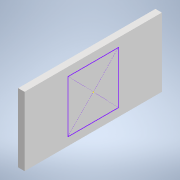
# Autodesk Inventor part: NASA-20-MM-MP-01
Saved by Autodesk Inventor 2020 (Build 240168000, 168)
## iProperties
Created: 2019-09-22
Part Number: NASA-20-MM-MP-01
Material: Aluminum 6061
Document SubType Name: Modeling
Designer: Rick Szalay
Density: 2.7 g/cm^3
Appearance: Aluminum - Flat
Author: Rick Szalay
Autodesk Inventor part; units mm, degrees
ref_plane "YZ Plane" through (0, 0, 0) normal (1, 0, 0) x (0, 1, 0)
ref_plane "XZ Plane" through (0, 0, 0) normal (0, 1, 0) x (-1, 0, 0)
ref_plane "XY Plane" through (0, 0, 0) normal (0, 0, 1) x (1, 0, 0)
sketch "Sketch1" plane through (0, 0, 0) normal (1, 0, 0) x (0, 1, 0)
  line L0 (-25.4, -50.8) -> (25.4, -50.8)
  line L1 (25.4, -50.8) -> (25.4, 50.8)
  line L2 (25.4, 50.8) -> (-25.4, 50.8)
  line L3 (-25.4, 50.8) -> (-25.4, -50.8)
  line L4 (-25.4, -50.8) -> (25.4, 50.8) construction
  line L5 (25.4, -50.8) -> (-25.4, 50.8) construction
  point P0 (0, 0)
  dimension "d0" = 50.8
  dimension "d1" = 101.6
  constraints: 12 end point, 2 midpoint, 2 parallel, 1 horizontal, 1 perpendicular
  measures "d0" distance of L0.start L0.end
  measures "d1" distance between parallel lines of L2 L0
extrude "Extrusion1" add sketch "Sketch1" along normal blind 57.15
fillet "Fillet2" radius 6.35 4 edges at (28.575, 25.4, 50.8) (28.575, -25.4, 50.8) (28.575, -25.4, -50.8) (28.575, 25.4, -50.8)
sketch "Sketch5" plane through (57.15, 0, 0) normal (1, 0, 0) x (0, 0, -1)
  arc A0 (50.8, 19.05) -> (44.45, 25.4) centre (44.45, 19.05) ccw projected
  line L0 (44.45, 25.4) -> (-44.45, 25.4) projected
  arc A1 (-44.45, 25.4) -> (-50.8, 19.05) centre (-44.45, 19.05) ccw projected
  line L1 (-50.8, 19.05) -> (-50.8, -19.05) projected
  arc A2 (-50.8, -19.05) -> (-44.45, -25.4) centre (-44.45, -19.05) ccw projected
  line L2 (-44.45, -25.4) -> (44.45, -25.4) projected
  arc A3 (44.45, -25.4) -> (50.8, -19.05) centre (44.45, -19.05) ccw projected
  line L3 (50.8, -19.05) -> (50.8, 19.05) projected
  point P0 (0, 0)
hole "Hole2" at (57.15, -19.05, -44.45) at (57.15, -19.05, 44.45) at (57.15, 19.05, 44.45) at (57.15, 19.05, -44.45) direction (-1, 0, 0) diameter 6.7564 end through all clearance for "Flat Head Machine Screw (82)" size "1/4" standard "Ansi Unified Screw Threads"
sketch "Sketch6" plane through (57.15, 0, 0) normal (1, 0, 0) x (0, 0, -1)
  circle A0 centre (44.45, -19.05) radius 3.3782 projected
  circle A1 centre (44.45, -19.05) radius 6.35
  circle A2 centre (44.45, 19.05) radius 3.3782 projected
  circle A3 centre (44.45, 19.05) radius 6.35
  circle A4 centre (-44.45, 19.05) radius 3.3782 projected
  circle A5 centre (-44.45, 19.05) radius 6.35
  circle A6 centre (-44.45, -19.05) radius 3.3782 projected
  circle A7 centre (-44.45, -19.05) radius 6.35
  line L0 (-46.99, 21.59) -> (46.99, 21.59)
  line L1 (46.99, 21.59) -> (46.99, -21.59)
  line L2 (46.99, -21.59) -> (-46.99, -21.59)
  line L3 (-46.99, -21.59) -> (-46.99, 21.59)
  line L4 (-46.99, 21.59) -> (46.99, -21.59) construction
  line L5 (46.99, 21.59) -> (-46.99, -21.59) construction
  arc A8 (44.45, -25.4) -> (50.8, -19.05) centre (44.45, -19.05) ccw projected
  arc A9 (50.8, 19.05) -> (44.45, 25.4) centre (44.45, 19.05) ccw projected
  arc A10 (-44.45, 25.4) -> (-50.8, 19.05) centre (-44.45, 19.05) ccw projected
  arc A11 (-50.8, -19.05) -> (-44.45, -25.4) centre (-44.45, -19.05) ccw projected
  line L6 (50.8, -19.05) -> (50.8, 19.05) projected
  point P0 (0, 0)
  point P1 (-46.99, 13.2301)
  point P2 (-46.99, -13.2301)
  point P3 (-38.6301, -21.59)
  point P4 (38.6301, -21.59)
  point P5 (46.99, -13.2301)
  point P6 (46.99, 13.2301)
  point P7 (38.6301, 21.59)
  point P8 (-38.6301, 21.59)
  dimension "d23" = 43.18
  dimension "d24" = 3.81
  constraints: 12 end point, 8 concentric, 4 centre point, 3 coincident, 2 midpoint, 2 parallel, 1 horizontal, 1 perpendicular
  measures "d23" distance of L0.end L1.end
  measures "d24" distance between parallel lines of L6 L1
extrude "Extrusion2" cut sketch "Sketch6" against normal through all contours A1 L2 A7 L3 A5 L0 A3 L1
fillet "Fillet3" radius 3.175 8 edges at (28.575, 13.2301, 46.99) (28.575, 21.59, 38.6301) (28.575, -21.59, -38.6301) (28.575, -13.2301, -46.99) (28.575, 13.2301, -46.99) (28.575, 21.59, -38.6301) (28.575, -21.59, 38.6301) (28.575, -13.2301, 46.99)
equation "\"d2\" = Base"
equation "\"Base\" = 57.15"
body "Solid1"
